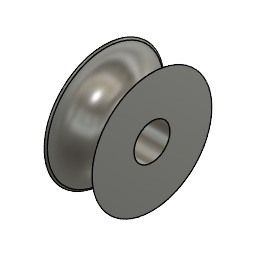
Pully (Autodesk Fusion 360 design; units mm, degrees)
part number: 2026-08-27-17-20-08-559
Autodesk Fusion 360 part; units mm, degrees
sketch "Sketch1" plane through (0, 0, 0) normal (1, 0, 0) x (0, 0, -1)
  circle A0 centre (0, 100) radius 50
  circle A1 centre (0, 100) radius 15
  dimension "d1" = 100
  dimension "d4" = 30
  constraint concentric A0 A1
  measures "d1" diameter of A0
  measures "d4" diameter of A1
extrude "Extrude1" add sketch "Sketch1" along normal mid plane 40
ref_plane "WorkPlane1" through (0.3689, 149.7557, -4.9371) normal (0, 0.098742, 0.995113) x (0, 0.995113, -0.098742)
sketch "Sketch2" plane through (0, 0.975, 9.826) normal (0, 0.098742, 0.995113) x (0, 0.995113, -0.098742)
sketch "Sketch3" plane through (0, 0.975, 9.826) normal (0, 0.098742, 0.995113) x (0, 0.995113, -0.098742)
  circle A0 centre (149.8, 0) radius 19
  dimension "d6" = 38
  measures "d6" diameter of A0
revolve "Revolve1" cut sketch "Sketch3" angle 360 about axis through (0, 100, 0) along (-1, 0, 0)
fillet "Fillet1" radius 2 2 edges at (-18.9978, 118.0808, 46.6164) (18.9978, 81.9192, 46.6164)
